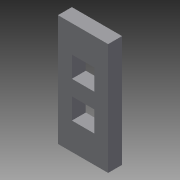
# Autodesk Inventor part: ShortSupportRod
Saved by Autodesk Inventor 2013 (Build 170138000, 138)
## iProperties
Created: 2013-01-18
Part Number: ShortSupportRod
Material: Generic
Document SubType Name: Modeling
Designer: motoennies
Density: 1 g/cm^3
Author: motoennies
Autodesk Inventor part; units mm, degrees
ref_plane "YZ Plane" through (0, 0, 0) normal (1, 0, 0) x (0, 1, 0)
ref_plane "XZ Plane" through (0, 0, 0) normal (0, 1, 0) x (-1, 0, 0)
ref_plane "XY Plane" through (0, 0, 0) normal (0, 0, 1) x (1, 0, 0)
sketch "Sketch1" plane through (0, 0, 0) normal (0, 0, 1) x (1, 0, 0)
  line L0 (0, 0) -> (0, 50.8)
  line L1 (0, 0) -> (22.86, 0)
  line L2 (22.86, 0) -> (22.86, 50.8)
  line L3 (22.86, 50.8) -> (0, 50.8)
  line L4 (6.35, 38.4048) -> (16.51, 38.4048)
  line L5 (6.35, 38.4048) -> (6.35, 28.8798)
  line L6 (6.35, 28.8798) -> (16.51, 28.8798)
  line L7 (16.51, 28.8798) -> (16.51, 38.4048)
  line L8 (0, 25.4) -> (22.86, 25.4) construction
  line L9 (6.35, 12.3952) -> (16.51, 12.3952)
  line L10 (6.35, 12.3952) -> (6.35, 21.9202)
  line L11 (6.35, 21.9202) -> (16.51, 21.9202)
  line L12 (16.51, 21.9202) -> (16.51, 12.3952)
  dimension "d0" = 50.8
  dimension "d1" = 22.86
  dimension "d2" = 10.16
  dimension "d3" = 12.3952
  dimension "d5" = 9.525
  dimension "d6" = 6.35
  constraints: 26 end point, 4 perpendicular, 4 symmetric about line, 3 parallel, 2 midpoint, 1 vertical
  measures "d0" distance of L0.start L0.end
  measures "d1" distance of L0.start L1.end
  measures "d2" distance of L4.start L4.end
  measures "d3" distance between parallel lines of L3 L4
  measures "d5" distance of L4.start L5.end
  measures "d6" distance between parallel lines of L2 L7
extrude "Extrusion1" add sketch "Sketch1" along normal blind 6.35
body "Solid1"
